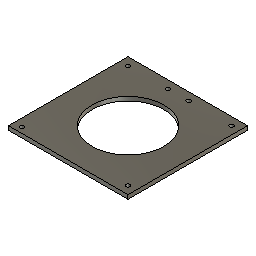
Thermoelectric Mist Cooler (Autodesk Fusion 360 design; units mm, degrees)
part number: 2026-07-06-14-47-51-385
Autodesk Fusion 360 part; units mm, degrees
sketch "Sketch1" plane through (0, 0, 0) normal (0, 0, 1) x (1, 0, 0)
  line L0 (0, 0) -> (150, 0)
  line L1 (150, 0) -> (150, 150)
  line L2 (150, 150) -> (0, 150)
  line L3 (0, 150) -> (0, 0)
  circle A0 centre (74.3636, 76.0684) radius 45
  dimension "d1" = 150
  dimension "d2" = 150
  dimension "d3" = 90
  constraint horizontal L0
  constraint vertical L1
  constraint horizontal L2
  constraint vertical L3
  constraint coincident L0.start L3.end
  measures "d1" distance of L0.start L0.end
  measures "d2" distance of L0.start L2.end
  measures "d3" diameter of A0
sketch "Sketch2" plane through (0, 0, 0) normal (0, 0, 1) x (1, 0, 0)
  circle A0 centre (11.6759, 139.6456) radius 2.5
  circle A1 centre (140, 140) radius 2.5
  circle A2 centre (10, 10) radius 2.5
  circle A3 centre (140, 10) radius 2.5
  circle A4 centre (60, 140) radius 2.5
  circle A5 centre (85.9996, 140.152) radius 2.5
  dimension "d4" = 5
  dimension "d5" = 5
  dimension "d6" = 5
  dimension "d7" = 5
  dimension "d8" = 5
  dimension "d9" = 5
  dimension "d10" = 26
  measures "d4" diameter of A0
  measures "d5" diameter of A1
  measures "d6" diameter of A2
  measures "d7" diameter of A3
  measures "d8" diameter of A4
  measures "d9" diameter of A5
  measures "d10" distance of A4.centre A5.centre
extrude "Extrude1" add sketch "Sketch1" sketch "Sketch2" along normal blind 5 contours L0 L1 L2 L3 | A0 of sketch 2
sketch "Sketch3" plane through (0, 0, 5) normal (0, 0, 1) x (-1, 0, 0)
  line L0 (0, -150) -> (0, 0)
  line L1 (0, 0) -> (-150, 0)
  line L2 (-150, 0) -> (-150, -150)
  line L3 (-150, -150) -> (0, -150)
  circle A0 centre (-75, -75) radius 45
  circle A1 centre (-10, -140) radius 2.5
  circle A2 centre (-140, -140) radius 2.5
  circle A3 centre (-10, -7) radius 2.5
  circle A4 centre (-140, -10) radius 2.5
  circle A5 centre (-60, -140) radius 2.5
  circle A6 centre (-86, -140) radius 2.5
  dimension "d13" = 90
  dimension "d14" = 75
  dimension "d15" = 75
  dimension "d16" = 5
  dimension "d17" = 5
  dimension "d18" = 5
  dimension "d19" = 5
  dimension "d20" = 5
  dimension "d21" = 5
  dimension "d22" = 26
  dimension "d23" = 133
  dimension "d24" = 130
  measures "d13" diameter of A0
  measures "d14" distance of L0 A0.centre
  measures "d15" distance of L3 A0.centre
  measures "d16" diameter of A1
  measures "d17" diameter of A2
  measures "d18" diameter of A3
  measures "d19" diameter of A4
  measures "d20" diameter of A5
  measures "d21" diameter of A6
  measures "d22" distance of A5.centre A6.centre
  measures "d23" distance of A1.centre A3.centre
  measures "d24" distance of A2.centre A4.centre
extrude "Extrude2" cut sketch "Sketch3" against normal blind 5 contours A0 | A1 | A2 | A3 | A4 | A5 | A6
